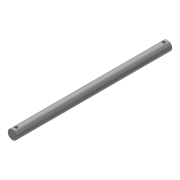
# Autodesk Inventor part: Handle_Rod
Saved by Autodesk Inventor 2022 (Build 260148000, 148)
## iProperties
Created: 2006-01-18
Part Number: Handle_Rod
Document SubType Name: Modeling
Designer: PMiller
Material: Steel, Mild
Density: 7.85 g/cm^3
Appearance: Steel
Mass: 49.4111 g
Surface Area: 34.334 cm^2
Volume: 6.29441 cm^3
Author: PMiller
Autodesk Inventor part; units mm, degrees
ref_plane "YZ Plane" through (0, 0, 0) normal (1, 0, 0) x (0, 1, 0)
ref_plane "XZ Plane" through (0, 0, 0) normal (0, 1, 0) x (-1, 0, 0)
ref_plane "XY Plane" through (0, 0, 0) normal (0, 0, 1) x (1, 0, 0)
sketch "Sketch1" plane through (0, 0, 0) normal (0, 0, 1) x (1, 0, 0)
  circle A0 centre (0, 0) radius 3.9497
  dimension "d0" = 7.8994
  constraints: 1 centre point, 1 coincident
  measures "d0" diameter of A0
extrude "Extrusion1" add sketch "Sketch1" against normal mid plane 130.175
sketch "Sketch2" plane through (0, 0, 0) normal (0, 1, 0) x (-1, 0, 0)
  circle A0 centre (0, 61.9125) radius 1.3208
  line L0 (-3.9497, 65.0875) -> (3.9497, 65.0875) projected
  point P0 (0, 65.0875)
  dimension "d3" = 2.6416
  dimension "d4" = 3.175
  constraints: 1 centre point, 1 midpoint, 1 vertical alignment
  measures "d3" diameter of A0
  measures "d4" distance from line of L0 A0.centre
extrude "Extrusion2" cut sketch "Sketch2" along normal through all both and the other way through all
mirror "Mirror1" about plane through (0, 0, 0) normal (0, 0, 1) of "Extrusion2"
body "Solid1"
